base_lamp v1 (Autodesk Fusion 360 design; units mm, degrees)
Autodesk Fusion 360 part; units mm, degrees
sketch "Boceto1" plane through (0, 0, 0) normal (0, 0, 1) x (1, 0, 0)
  circle A0 centre (0, 0) radius 50
  dimension "d4" = 100
  constraint coincident A0.centre origin
  measures "d4" diameter of A0
extrude "Extruir1" add sketch "Boceto1" along normal blind 60
sketch "Boceto2" plane through (0, 0, 60) normal (0, 0, 1) x (-1, 0, 0)
  circle A0 centre (0, 0) radius 50
  circle A1 centre (0, 0) radius 47.5
  circle A2 centre (0, 0) radius 42.5
  circle A3 centre (0, 0) radius 40
  dimension "d7" = 95
  dimension "d8" = 85
  dimension "d9" = 80
  constraint concentric A0 A1
  constraint coincident A0.centre A1.centre
  constraint concentric A2 A3
  measures "d7" diameter of A1
  measures "d8" diameter of A2
  measures "d9" diameter of A3
extrude "Extruir2" cut sketch "Boceto2" against normal blind 5 contours A1 | A3
extrude "Extruir3" cut 1 faces at (-12.741, 3.9301, 55) along direction (0, 0, -1) blind 50
sketch "Boceto3" plane through (0, 0, 5) normal (0, 0, 1) x (-1, 0, 0)
  circle A0 centre (0, 0) radius 45
  dimension "d14" = 90
  measures "d14" diameter of A0
extrude "Extruir4" cut sketch "Boceto3" along normal blind 47
equation "DiametroBase = 100 mm"
equation "AlturaBase = 60 mm"
equation "AlturaPantalla = 200 mm"
equation "d4 = DiametroBase"
equation "d5 = AlturaBase"
named bodies: "Base"
